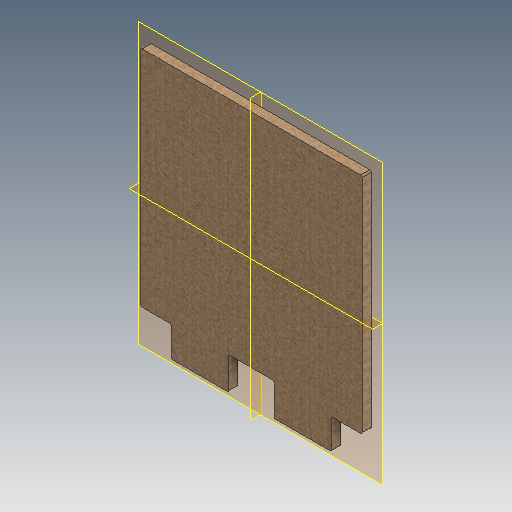
# Autodesk Inventor part: MDF_Front_Side
Saved by Autodesk Inventor 2021 (Build 250183000, 183)
## iProperties
Created: 2021-02-17
Part Number: MDF_Front_Side
Material: MDF Medium Density Fiberboard
Document SubType Name: Modeling
Designer: negt20
Density: 0.8 g/cm^3
Appearance: Cardboard - Corrugated
Author: negt20
Autodesk Inventor part; units mm, degrees
sketch "Sketch1" plane through (0, 0, 0) normal (0, 0, 1) x (1, 0, 0)
  line L0 (-73, 83.75) -> (73, 83.75)
  line L1 (73, 83.75) -> (73, -83.75)
  line L2 (73, -83.75) -> (-73, -83.75)
  line L3 (-73, -83.75) -> (-73, 83.75)
  point P0 (0, 83.75)
  point P1 (0, 0)
  point P2 (-73, 0)
  dimension "d0" = 146
  dimension "d1" = 167.5
  constraints: 8 end point, 2 midpoint, 2 parallel, 1 horizontal, 1 horizontal alignment, 1 perpendicular, 1 vertical alignment
  measures "d0" distance of L1.end L2.end
  measures "d1" distance of L0.end L1.end
extrude "Extrusion1" add sketch "Sketch1" along normal blind 6
sketch "Sketch2" plane through (0, 0, 6) normal (0, 0, 1) x (1, 0, 0)
  line L0 (-73, 83.75) -> (-73, -83.75) projected
  line L1 (-73, -83.75) -> (-73, -63.75)
  line L2 (-67.5, -78.25) -> (-53, -78.25)
  line L3 (-53, -78.25) -> (-53, -83.75)
  line L4 (-73, -63.75) -> (-53, -63.75)
  line L5 (-53, -63.75) -> (-53, -83.75)
  line L6 (-73, -83.75) -> (73, -83.75) projected
  line L7 (-53, -83.75) -> (-73, -83.75)
  point P0 (0, 0)
  point P1 (40.5, -62.5)
  dimension "d14" = 20
  dimension "d18" = 20
  constraints: 12 end point, 2 perpendicular, 1 collinear, 1 horizontal, 1 point on line
  measures "d14" distance of L0.end L1.end
  measures "d18" distance of L1.end L4.end
extrude "Extrusion2" cut sketch "Sketch2" against normal blind 6
mirror "Mirror1" about plane through (0, 0, 0) normal (1, 0, 0) of "Extrusion2"
sketch "Sketch4" plane through (0, 0, 0) normal (0, 0, -1) x (-1, 0, 0)
  line L0 (-15, -62.25) -> (15, -62.25)
  line L1 (15, -62.25) -> (15, -83.75)
  line L2 (15, -83.75) -> (-15, -83.75)
  line L3 (-15, -83.75) -> (-15, -62.25)
  line L4 (53, -83.75) -> (-53, -83.75) projected
  point P0 (0, 0)
  point P1 (0, -83.75)
  point P2 (0, -83.75)
  point P3 (0, -83.75)
  dimension "d19" = 30
  dimension "d20" = 21.5
  constraints: 8 end point, 3 midpoint, 2 coincident, 2 parallel, 1 horizontal, 1 perpendicular
  measures "d19" distance of L1.end L2.end
  measures "d20" distance of L0.end L1.end
extrude "Extrusion4" cut sketch "Sketch4" against normal blind 6
fillet "Fillet1" radius 1 12 edges at (73, -63.75, 3) (53, -63.75, 3) (53, -83.75, 3) (15, -83.75, 3) (-15, -83.75, 3) (-15, -62.25, 3) (-53, -83.75, 3) (15, -62.25, 3) (-53, -63.75, 3) (-73, -63.75, 3) (-73, 83.75, 3) (73, 83.75, 3)
body "Solid1"
